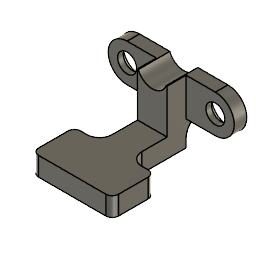
cableHolder (Autodesk Fusion 360 design; units mm, degrees)
Autodesk Fusion 360 part; units mm, degrees
note: some values were not read from the file. Set by a fixed rule: which sketch regions a step uses.
sketch "Sketch1" plane through (0, 0, 0) normal (0, 0, 1) x (1, 0, 0)
  line L0 (-5.35, 0) -> (5.35, 0)
  line L1 (6.35, 1) -> (6.35, 5.7)
  line L2 (-6.35, 5.7) -> (-6.35, 1)
  line L3 (2.35, 8.7) -> (2.35, 15.7)
  line L4 (2.35, 15.7) -> (-2.35, 15.7)
  line L5 (-2.35, 15.7) -> (-2.35, 8.7)
  line L6 (5.35, 6.7) -> (4.35, 6.7)
  line L7 (-4.35, 6.7) -> (-5.35, 6.7)
  arc A0 (-5.35, 6.7) -> (-6.35, 5.7) centre (-5.35, 5.7) ccw
  arc A1 (-6.35, 1) -> (-5.35, 0) centre (-5.35, 1) ccw
  arc A2 (5.35, 0) -> (6.35, 1) centre (5.35, 1) ccw
  arc A3 (6.35, 5.7) -> (5.35, 6.7) centre (5.35, 5.7) ccw
  arc A4 (2.35, 8.7) -> (4.35, 6.7) centre (4.35, 8.7) ccw
  arc A5 (-4.35, 6.7) -> (-2.35, 8.7) centre (-4.35, 8.7) ccw
  point P0 (6.35, 0)
  point P1 (6.35, 6.7)
  point P2 (-2.35, 6.7)
  dimension "d1" = 6.35
  dimension "d2" = 12.7
  dimension "d3" = 6.7
  dimension "d4" = 9
  dimension "d5" = 4.7
  dimension "d6" = 2.35
  dimension "d26" = 2
  dimension "d27" = 2
  dimension "d28" = 1
  dimension "d29" = 1
  dimension "d30" = 1
  dimension "d31" = 1
  constraint horizontal L0
  constraint vertical L1
  constraint horizontal L6
  constraint vertical L2
  constraint vertical L3
  constraint horizontal L4
  constraint vertical L5
  constraint coincident P2 L6
  constraint collinear L6 L7
  constraint horizontal origin P0
  constraint coincident P2 L5
  constraint tangent L2 A0
  constraint tangent L7 A0
  constraint tangent L0 A1
  constraint tangent L2 A1
  constraint coincident P0 L0
  constraint coincident P0 L1
  constraint tangent L0 A2
  constraint tangent L1 A2
  constraint coincident P1 L1
  constraint coincident P1 L6
  constraint tangent L1 A3
  constraint tangent L6 A3
  constraint tangent L3 A4
  constraint tangent L6 A4
  constraint vertical L7.start A5.centre
  constraint coincident L7.start A5.start
  constraint tangent L5 A5
  measures "d1" distance of origin L1
  measures "d2" distance of L1 L2
  measures "d3" distance of P0 P1
  measures "d4" distance of P2 L4.end
  measures "d5" distance of L3.end L4.end
  measures "d6" horizontal distance of origin L3.end
  measures "d26" radius of A5
  measures "d27" radius of A4
  measures "d28" radius of A3
  measures "d29" radius of A2
  measures "d30" radius of A1
  measures "d31" radius of A0
extrude "Extrude1" add sketch "Sketch1" along normal blind 3
sketch "Sketch2" plane through (0, 15.7, 0) normal (0, 1, 0) x (-1, 0, 0)
  line L0 (-2.35, 0) -> (2.35, 0)
  line L1 (2.35, 0) -> (2.35, 3)
  line L2 (2.35, 3) -> (-2.35, 3)
  line L3 (-2.35, 3) -> (-2.35, 0)
  line L4 (-2.35, 3) -> (2.35, 3)
  line L5 (2.35, 3) -> (2.35, 10.8)
  line L6 (2.35, 10.8) -> (-2.35, 10.8)
  line L7 (-2.35, 10.8) -> (-2.35, 3)
  circle A0 centre (0, 10.8) radius 2.35
  line L8 (-2.35, 10) -> (2.35, 10)
  dimension "d10" = 4.7
  dimension "d11" = 7.8
  dimension "d22" = 7
  constraint horizontal L4
  constraint vertical L5
  constraint horizontal L6
  constraint vertical L7
  constraint coincident L2.end L3.start
  constraint midpoint L6 A0.centre
  constraint coincident L5.end A0
  constraint coincident L7 L8.start
  constraint coincident L5 L8.end
  constraint perpendicular L5 L8
  measures "d10" distance of L2.end L1.end
  measures "d11" distance of L2.end L6.end
  measures "d22" distance of L2.end L8
extrude "Extrude2" add sketch "Sketch2" against normal blind 3 contours L2 L4 L5 L7 A0 L8
sketch "Sketch3" plane through (0, 15.7, 0) normal (0, 1, 0) x (-1, 0, 0)
  line L0 (-2.35, 0) -> (2.35, 0)
  line L1 (2.35, 0) -> (2.35, 10)
  arc A0 (-2.2096, 10) -> (2.2096, 10) centre (0, 10.8) ccw
  line L2 (-2.35, 10) -> (-2.35, 0)
  circle A1 centre (-7, 7) radius 1.5
  circle A2 centre (7, 7) radius 1.5
  line L3 (-7, 4) -> (7, 4)
  arc A3 (7, 4) -> (7, 10) centre (7, 7) ccw
  line L4 (7, 10) -> (-7, 10)
  arc A4 (-7, 10) -> (-7, 4) centre (-7, 7) ccw
  line L5 (-7, 7) -> (7, 7) construction
  line L6 (2.35, 10) -> (2.2096, 10)
  line L7 (-2.2096, 10) -> (-2.35, 10)
  dimension "d14" = 3
  dimension "d15" = 3
  dimension "d16" = 7
  dimension "d17" = 14
  dimension "d18" = 7
  dimension "d19" = 6
  constraint horizontal A1.centre A2.centre
  constraint tangent L3 A3
  constraint tangent A3 L4
  constraint parallel L3 L4
  constraint tangent L4 A4
  constraint tangent L3 A4
  constraint coincident A2.centre A3.centre
  constraint perpendicular L1 L5
  constraint coincident A1.centre A4.centre
  measures "d14" diameter of A1
  measures "d15" diameter of A2
  measures "d16" vertical distance of origin A1.centre
  measures "d17" distance of A1.centre A2.centre
  measures "d18" horizontal distance of origin A1.centre
  measures "d19" diameter of A3
extrude "Extrude3" add sketch "Sketch3" along normal blind 2 contours L2 L3 L4 A4 | L1 A0 L2 L3 L4 L6 L7 | L1 L3 A3 L4
fillet "Fillet1" radius 3 1 edges at (0, 15.7, 4)
chamfer "Chamfer1" distance 1.1 angle 45 2 edges at (8.3985, 17.7, 7.5424) (-5.6015, 17.7, 7.5424)
equation "d1 = ( ( 13 - 0.3 ) / 2 ) * 1 mm"
equation "d2 = 13 mm - 0.3 mm"
equation "d3 = 7 mm - 0.3 mm"
equation "d6 = ( 4.7 / 2 ) * 1 mm"
